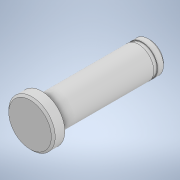
# Autodesk Inventor part: Bolt
Saved by Autodesk Inventor 2022 (Build 260153000, 153)
## iProperties
Created: 2021-12-04
Part Number: Bolt
Material: Generic
Document SubType Name: Modeling
Designer: LEGION SMIT
Density: 1 g/cm^3
Appearance: Default
Author: LEGION SMIT
Autodesk Inventor part; units mm, degrees
ref_plane "YZ Plane" through (0, 0, 0) normal (1, 0, 0) x (0, 1, 0)
ref_plane "XZ Plane" through (0, 0, 0) normal (0, 1, 0) x (-1, 0, 0)
ref_plane "XY Plane" through (0, 0, 0) normal (0, 0, 1) x (1, 0, 0)
sketch "Sketch1" plane through (0, 0, 0) normal (0, 0, 1) x (1, 0, 0)
  circle A0 centre (0, 0) radius 6
  dimension "d0" = 12
  constraints: 1 centre point, 1 coincident
  measures "d0" diameter of A0
extrude "Extrusion1" add sketch "Sketch1" against normal blind 3
chamfer "Chamfer1" distance 0.5 angle 45 1 edges at (-6, 0, 0) measured on face at (5.9805, -0.4828, -2)
sketch "Sketch2" plane through (0, 0, -3) normal (0, 0, -1) x (-1, 0, 0)
  circle A0 centre (0, 0) radius 4
  dimension "d6" = 8
  constraints: 1 centre point, 1 coincident
  measures "d6" diameter of A0
extrude "Extrusion2" add sketch "Sketch2" along normal blind 25
sketch "Sketch3" plane through (0, 0, -28) normal (0, 0, -1) x (-1, 0, 0)
  circle A0 centre (0, 0) radius 3.8
  dimension "d9" = 7.6
  constraints: 1 centre point, 1 coincident
  measures "d9" diameter of A0
extrude "Extrusion3" add sketch "Sketch3" along normal blind 1
sketch "Sketch4" plane through (0, 0, -29) normal (0, 0, -1) x (-1, 0, 0)
  circle A0 centre (0, 0) radius 4
  constraints: 1 centre point, 1 coincident
extrude "Extrusion4" add sketch "Sketch4" along normal blind 2
chamfer "Chamfer2" distance 0.5 angle 45 1 edges at (4, 0, -31)
body "Solid1"
